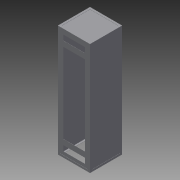
# Autodesk Inventor part: Cabinet_2x2x7
Saved by Autodesk Inventor 2013 SP2 (Build 170200200, 200)
## iProperties
Created: 2015-04-30
Part Number: Cabinet_2x2x7
Material: Generic
Document SubType Name: Modeling
Designer: mcgratta
Density: 1 g/cm^3
Author: mcgratta
Autodesk Inventor part; units mm, degrees
ref_plane "YZ Plane" through (0, 0, 0) normal (1, 0, 0) x (0, 1, 0)
ref_plane "XZ Plane" through (0, 0, 0) normal (0, 1, 0) x (-1, 0, 0)
sketch "Sketch1" plane through (0, 0, 0) normal (0, 1, 0) x (-1, 0, 0)
  line L0 (0, 0) -> (-615.95, 0)
  line L1 (-615.95, 0) -> (-615.95, -615.95)
  line L2 (-615.95, -615.95) -> (0, -615.95)
  line L3 (0, -615.95) -> (0, 0)
  line L4 (-38.1, -38.1) -> (-577.85, -38.1)
  line L5 (-577.85, -38.1) -> (-577.85, -577.85)
  line L6 (-577.85, -577.85) -> (-38.1, -577.85)
  line L7 (-38.1, -577.85) -> (-38.1, -38.1)
  dimension "d0" = 615.95
  dimension "d2" = 615.95
  dimension "d3" = 38.1
  dimension "d4" = 38.1
  dimension "d5" = 38.1
  dimension "d6" = 38.1
  constraints: 16 end point, 4 parallel, 2 horizontal, 2 perpendicular
  measures "d0" distance between parallel lines of L1 L3
  measures "d2" distance between parallel lines of L0 L2
  measures "d3" distance between parallel lines of L4 L0
  measures "d4" distance between parallel lines of L6 L2
  measures "d5" distance between parallel lines of L7 L3
  measures "d6" distance between parallel lines of L1 L5
extrude "Extrusion1" add sketch "Sketch1" along normal blind 3.175
sketch "Sketch2" plane through (0, 3.175, 0) normal (0, 1, 0) x (1, 0, 0)
  line L0 (0, 0) -> (615.95, 0) projected
  line L1 (615.95, 0) -> (615.95, 615.95) projected
  line L2 (0, 0) -> (615.95, 0)
  line L3 (615.95, 0) -> (615.95, 615.95)
  line L4 (615.95, 615.95) -> (0, 615.95)
  line L5 (0, 615.95) -> (0, 0)
  line L6 (3.175, 3.175) -> (612.775, 3.175)
  line L7 (612.775, 3.175) -> (612.775, 612.775)
  line L8 (612.775, 612.775) -> (3.175, 612.775)
  line L9 (3.175, 612.775) -> (3.175, 3.175)
  dimension "d9" = 3.175
  dimension "d11" = 3.175
  dimension "d12" = 3.175
  dimension "d13" = 3.175
  constraints: 16 end point, 4 parallel, 2 horizontal, 2 perpendicular
  measures "d9" distance between parallel lines of L9 L5
  measures "d11" distance between parallel lines of L0 L6
  measures "d12" distance between parallel lines of L1 L7
  measures "d13" distance between parallel lines of L4 L8
extrude "Extrusion2" add sketch "Sketch2" along normal blind 34.925
sketch "Sketch3" plane through (0, 38.1, 0) normal (0, 1, 0) x (1, 0, 0)
  line L0 (3.175, 3.175) -> (3.175, 612.775) projected
  line L1 (612.775, 3.175) -> (3.175, 3.175) projected
  line L2 (0, 0) -> (615.95, 0) projected
  line L3 (0, 615.95) -> (0, 0) projected
  line L4 (3.175, 3.175) -> (3.175, 38.1)
  line L5 (0, 38.1) -> (0, 0)
  line L6 (38.1, 0) -> (38.1, 3.175)
  line L7 (0, 38.1) -> (3.175, 38.1)
  dimension "d16" = 38.1
  dimension "d17" = 38.1
  dimension "d18" = 38.1
  constraints: 8 end point, 4 point on line, 1 collinear, 1 perpendicular
  measures "d16" distance between parallel lines of L5 L6
  measures "d17" distance from line of L2 L5.start
  measures "d18" distance from line of L2 L4.end
extrude "Extrusion3" add sketch "Sketch3" along normal blind 2063.75
sketch "Sketch4" plane through (0, 38.1, 0) normal (0, 1, 0) x (1, 0, 0)
  line L0 (612.775, 612.775) -> (612.775, 3.175) projected
  line L1 (612.775, 3.175) -> (38.1, 3.175) projected
  line L2 (38.1, 0) -> (615.95, 0) projected
  line L3 (615.95, 0) -> (615.95, 615.95) projected
  line L4 (612.775, 3.175) -> (577.85, 3.175)
  line L5 (577.85, 0) -> (615.95, 0)
  line L6 (615.95, 38.1) -> (612.775, 38.1)
  line L7 (577.85, 0) -> (577.85, 3.175)
  point P0 (0, 0)
  dimension "d21" = 38.1
  dimension "d22" = 38.1
  dimension "d23" = 34.925
  constraints: 8 end point, 4 point on line, 1 collinear, 1 perpendicular
  measures "d21" distance between parallel lines of L5 L6
  measures "d22" distance of L5.start L2.end
  measures "d23" distance of L4.end L0.end
extrude "Extrusion4" add sketch "Sketch4" along normal blind 2063.75
sketch "Sketch5" plane through (0, 38.1, 0) normal (0, 1, 0) x (1, 0, 0)
  line L0 (615.95, 38.1) -> (615.95, 615.95) projected
  line L1 (615.95, 615.95) -> (0, 615.95) projected
  line L2 (3.175, 612.775) -> (612.775, 612.775) projected
  line L3 (612.775, 612.775) -> (612.775, 38.1) projected
  line L4 (612.775, 612.775) -> (577.85, 612.775)
  line L5 (577.85, 615.95) -> (615.95, 615.95)
  line L6 (615.95, 577.85) -> (612.775, 577.85)
  line L7 (577.85, 612.775) -> (577.85, 615.95)
  point P0 (0, 0)
  dimension "d26" = 38.1
  dimension "d27" = 38.1
  dimension "d28" = 38.1
  constraints: 8 end point, 4 point on line, 1 collinear, 1 perpendicular
  measures "d26" distance of L0.end L5.start
  measures "d27" distance from line of L0 L4.end
  measures "d28" distance between parallel lines of L1 L6
extrude "Extrusion5" add sketch "Sketch5" along normal blind 2063.75
sketch "Sketch6" plane through (0, 38.1, 0) normal (0, 1, 0) x (1, 0, 0)
  line L0 (577.85, 615.95) -> (0, 615.95) projected
  line L1 (0, 615.95) -> (0, 38.1) projected
  line L2 (3.175, 38.1) -> (3.175, 612.775) projected
  line L3 (3.175, 612.775) -> (577.85, 612.775) projected
  line L4 (0, 615.95) -> (0, 577.85)
  line L5 (3.175, 577.85) -> (3.175, 612.775)
  line L6 (38.1, 612.775) -> (38.1, 615.95)
  line L7 (0, 577.85) -> (3.175, 577.85)
  point P0 (0, 0)
  dimension "d31" = 38.1
  dimension "d32" = 38.1
  dimension "d33" = 38.1
  constraints: 8 end point, 4 point on line, 1 collinear, 1 perpendicular
  measures "d31" distance between parallel lines of L6 L4
  measures "d32" distance from line of L4.end L0
  measures "d33" distance from line of L5.start L0
extrude "Extrusion6" add sketch "Sketch6" along normal blind 2063.75
sketch "Sketch7" plane through (0, 3.175, 0) normal (0, 1, 0) x (1, 0, 0)
  line L0 (3.175, 612.775) -> (3.175, 3.175) projected
  line L1 (3.175, 612.775) -> (5.8318, 612.775)
  line L2 (5.8318, 612.775) -> (5.8318, 3.175)
  line L3 (5.8318, 3.175) -> (3.175, 3.175)
  line L4 (3.175, 3.175) -> (3.175, 612.775)
  point P0 (0, 0)
  dimension "d36" = 609.6
  dimension "d38" = 2.6568
  constraints: 8 end point, 2 parallel, 1 horizontal, 1 perpendicular
  measures "d36" distance between parallel lines of L1 L3
  measures "d38" distance between parallel lines of L2 L0
extrude "Extrusion7" add sketch "Sketch7" along normal blind 2133.6
sketch "Sketch8" plane through (0, 3.175, 0) normal (0, 1, 0) x (1, 0, 0)
  line L0 (612.775, 3.175) -> (612.775, 612.775) projected
  line L1 (612.775, 612.775) -> (610.1182, 612.775)
  line L2 (610.1182, 612.775) -> (610.1182, 3.175)
  line L3 (610.1182, 3.175) -> (612.775, 3.175)
  line L4 (612.775, 3.175) -> (612.775, 612.775)
  point P0 (0, 0)
  dimension "d41" = 609.6
  dimension "d43" = 2.6568
  constraints: 8 end point, 2 parallel, 1 horizontal, 1 perpendicular
  measures "d41" distance between parallel lines of L1 L3
  measures "d43" distance between parallel lines of L0 L2
extrude "Extrusion8" add sketch "Sketch8" along normal blind 2133.6
sketch "Sketch9" plane through (0, 3.175, 0) normal (0, 1, 0) x (1, 0, 0)
  line L0 (610.1182, 612.775) -> (5.8318, 612.775) projected
  line L1 (5.8318, 612.775) -> (610.1182, 612.775)
  line L2 (610.1182, 612.775) -> (610.1182, 610.1182)
  line L3 (610.1182, 610.1182) -> (5.8318, 610.1182)
  line L4 (5.8318, 610.1182) -> (5.8318, 612.775)
  point P0 (0, 0)
  dimension "d46" = 604.2863
  dimension "d48" = 2.6568
  constraints: 8 end point, 2 parallel, 1 horizontal, 1 perpendicular
  measures "d46" distance between parallel lines of L2 L4
  measures "d48" distance between parallel lines of L3 L0
extrude "Extrusion9" add sketch "Sketch9" along normal blind 2133.6
sketch "Sketch10" plane through (0, 3.175, 0) normal (0, 1, 0) x (1, 0, 0)
  line L0 (5.8318, 3.175) -> (610.1182, 3.175) projected
  line L1 (5.8318, 3.175) -> (610.1182, 3.175)
  line L2 (610.1182, 3.175) -> (610.1182, 5.8318)
  line L3 (610.1182, 5.8318) -> (5.8318, 5.8318)
  line L4 (5.8318, 5.8318) -> (5.8318, 3.175)
  point P0 (0, 0)
  dimension "d51" = 604.2863
  dimension "d53" = 2.6568
  constraints: 8 end point, 2 parallel, 1 horizontal, 1 perpendicular
  measures "d51" distance between parallel lines of L2 L4
  measures "d53" distance between parallel lines of L0 L3
extrude "Extrusion10" add sketch "Sketch10" along normal blind 2133.6
sketch "Sketch11" plane through (0, 2101.85, 0) normal (0, 1, 0) x (1, 0, 0)
  line L0 (577.85, 0) -> (615.95, 0) projected
  line L1 (612.775, 38.1) -> (612.775, 3.175) projected
  line L2 (615.95, 0) -> (0, 0)
  line L3 (0, 0) -> (0, 615.95)
  line L4 (0, 615.95) -> (615.95, 615.95)
  line L5 (615.95, 615.95) -> (615.95, 0)
  line L6 (612.775, 3.175) -> (3.175, 3.175)
  line L7 (3.175, 3.175) -> (3.175, 612.775)
  line L8 (3.175, 612.775) -> (612.775, 612.775)
  line L9 (612.775, 612.775) -> (612.775, 3.175)
  point P0 (0, 0)
  dimension "d56" = 615.95
  dimension "d58" = 615.95
  dimension "d59" = 609.6
  dimension "d60" = 609.6
  constraints: 16 end point, 4 parallel, 2 horizontal, 2 perpendicular
  measures "d56" distance between parallel lines of L5 L3
  measures "d58" distance between parallel lines of L4 L0
  measures "d59" distance between parallel lines of L6 L8
  measures "d60" distance between parallel lines of L1 L7
extrude "Extrusion11" add sketch "Sketch11" along normal blind 38.1
sketch "Sketch12" plane through (0, 2136.775, 0) normal (0, 1, 0) x (1, 0, 0)
  line L0 (3.175, 612.775) -> (3.175, 3.175) projected
  line L1 (3.175, 612.775) -> (612.775, 612.775)
  line L2 (612.775, 612.775) -> (612.775, 3.175)
  line L3 (612.775, 3.175) -> (3.175, 3.175)
  line L4 (3.175, 3.175) -> (3.175, 612.775)
  line L5 (38.1, 577.85) -> (577.85, 577.85)
  line L6 (577.85, 577.85) -> (577.85, 38.1)
  line L7 (577.85, 38.1) -> (38.1, 38.1)
  line L8 (38.1, 38.1) -> (38.1, 577.85)
  line L9 (0, 615.95) -> (0, 0) projected
  line L10 (615.95, 615.95) -> (0, 615.95) projected
  dimension "d63" = 609.6
  dimension "d65" = 609.6
  dimension "d66" = 38.1
  dimension "d67" = 38.1
  dimension "d68" = 539.75
  dimension "d69" = 539.75
  constraints: 16 end point, 4 parallel, 2 horizontal, 2 perpendicular
  measures "d63" distance between parallel lines of L3 L1
  measures "d65" distance between parallel lines of L2 L0
  measures "d66" distance between parallel lines of L8 L9
  measures "d67" distance between parallel lines of L5 L10
  measures "d68" distance between parallel lines of L6 L8
  measures "d69" distance between parallel lines of L7 L5
extrude "Extrusion12" add sketch "Sketch12" along normal blind 3.175
ref_plane "Work Plane1" through (0, 2134.1182, 0) normal (0, 1, 0) x (1, 0, 0)
sketch "Sketch13" plane through (0, 2134.1182, 0) normal (0, 1, 0) x (1, 0, 0)
  line L0 (5.8318, 5.8318) -> (610.1182, 5.8318)
  line L1 (610.1182, 5.8318) -> (610.1182, 610.1182)
  line L2 (610.1182, 610.1182) -> (5.8318, 610.1182)
  line L3 (5.8318, 610.1182) -> (5.8318, 5.8318)
  line L4 (0, 0) -> (615.95, 0) projected
  line L5 (0, 615.95) -> (0, 0) projected
  dimension "d73" = 5.8318
  dimension "d74" = 5.8318
  dimension "d75" = 604.2863
  dimension "d76" = 604.2863
  constraints: 8 end point, 2 parallel, 1 horizontal, 1 perpendicular
  measures "d73" distance between parallel lines of L4 L0
  measures "d74" distance between parallel lines of L5 L3
  measures "d75" distance between parallel lines of L1 L3
  measures "d76" distance between parallel lines of L2 L0
extrude "Extrusion13" add sketch "Sketch13" along normal blind 2.6568
sketch "Sketch14" plane through (38.1, 38.1, -3.175) normal (0, 0, 1) x (1, 0, 0)
  line L0 (539.75, 2063.75) -> (0, 2063.75) projected
  line L1 (0, 0) -> (0, 2063.75) projected
  line L2 (539.75, 0) -> (0, 0) projected
  line L3 (539.75, 0) -> (539.75, 2063.75) projected
  line L4 (63.5, 2000.25) -> (476.25, 2000.25)
  line L5 (476.25, 2000.25) -> (476.25, 1898.65)
  line L6 (476.25, 1898.65) -> (63.5, 1898.65)
  line L7 (63.5, 1898.65) -> (63.5, 2000.25)
  line L8 (63.5, 1797.05) -> (476.25, 1797.05)
  line L9 (476.25, 1797.05) -> (476.25, 266.7)
  line L10 (476.25, 266.7) -> (63.5, 266.7)
  line L11 (63.5, 266.7) -> (63.5, 1797.05)
  line L12 (63.5, 165.1) -> (476.25, 165.1)
  line L13 (476.25, 165.1) -> (476.25, 63.5)
  line L14 (476.25, 63.5) -> (63.5, 63.5)
  line L15 (63.5, 63.5) -> (63.5, 165.1)
  point P0 (-38.1, -38.1)
  dimension "d79" = 63.5
  dimension "d80" = 63.5
  dimension "d81" = 63.5
  dimension "d82" = 101.6
  dimension "d83" = 101.6
  dimension "d84" = 0
  dimension "d85" = 0
  dimension "d86" = 63.5
  dimension "d87" = 101.6
  dimension "d88" = 101.6
  dimension "d89" = 0
  dimension "d90" = 0
  constraints: 24 end point, 6 parallel, 3 horizontal, 3 perpendicular
  measures "d79" distance between parallel lines of L11 L1
  measures "d80" distance between parallel lines of L3 L9
  measures "d81" distance between parallel lines of L4 L0
  measures "d82" distance between parallel lines of L6 L4
  measures "d83" distance between parallel lines of L8 L6
  measures "d84" distance between parallel lines of L11 L7
  measures "d85" distance between parallel lines of L9 L5
  measures "d86" distance between parallel lines of L14 L2
  measures "d87" distance between parallel lines of L12 L10
  measures "d88" distance between parallel lines of L14 L12
  measures "d89" distance between parallel lines of L11 L15
  measures "d90" distance between parallel lines of L9 L13
extrude "Extrusion14" cut sketch "Sketch14" against normal blind 2.6568 contours L4 L5 L6 L7 | L8 L9 L10 L11 | L12 L13 L14 L15
sketch "Sketch15" plane through (577.85, 38.1, -612.775) normal (0, 0, -1) x (-1, 0, 0)
  line L0 (539.75, 2063.75) -> (0, 2063.75) projected
  line L1 (0, 0) -> (0, 2063.75) projected
  line L2 (539.75, 0) -> (0, 0) projected
  line L3 (539.75, 0) -> (539.75, 2063.75) projected
  line L4 (63.5, 2000.25) -> (476.25, 2000.25)
  line L5 (476.25, 2000.25) -> (476.25, 1898.65)
  line L6 (476.25, 1898.65) -> (63.5, 1898.65)
  line L7 (63.5, 1898.65) -> (63.5, 2000.25)
  line L8 (63.5, 1797.05) -> (476.25, 1797.05)
  line L9 (476.25, 1797.05) -> (476.25, 266.7)
  line L10 (476.25, 266.7) -> (63.5, 266.7)
  line L11 (63.5, 266.7) -> (63.5, 1797.05)
  line L12 (63.5, 165.1) -> (476.25, 165.1)
  line L13 (476.25, 165.1) -> (476.25, 63.5)
  line L14 (476.25, 63.5) -> (63.5, 63.5)
  line L15 (63.5, 63.5) -> (63.5, 165.1)
  point P0 (577.85, -38.1)
  dimension "d93" = 63.5
  dimension "d94" = 63.5
  dimension "d95" = 63.5
  dimension "d96" = 101.6
  dimension "d97" = 101.6
  dimension "d98" = 0
  dimension "d99" = 0
  dimension "d100" = 101.6
  dimension "d101" = 101.6
  dimension "d102" = 63.5
  dimension "d103" = 0
  dimension "d104" = 0
  constraints: 24 end point, 6 parallel, 3 horizontal, 3 perpendicular
  measures "d93" distance between parallel lines of L11 L1
  measures "d94" distance between parallel lines of L3 L9
  measures "d95" distance between parallel lines of L4 L0
  measures "d96" distance between parallel lines of L8 L6
  measures "d97" distance between parallel lines of L6 L4
  measures "d98" distance between parallel lines of L11 L7
  measures "d99" distance between parallel lines of L9 L5
  measures "d100" distance between parallel lines of L12 L10
  measures "d101" distance between parallel lines of L14 L12
  measures "d102" distance between parallel lines of L2 L14
  measures "d103" distance between parallel lines of L11 L15
  measures "d104" distance between parallel lines of L9 L13
extrude "Extrusion15" cut sketch "Sketch15" against normal blind 2.6568 contours L4 L5 L6 L7 | L8 L9 L10 L11 | L12 L13 L14 L15
body "Solid1"
